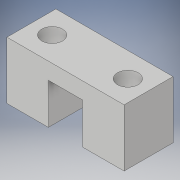
# Autodesk Inventor part: motor mount
Saved by Autodesk Inventor 2018 (Build 220112000, 112)
## iProperties
Created: 2019-04-09
Part Number: motor mount
Material: Generic
Document SubType Name: Modeling
Designer: Jayden
Density: 1 g/cm^3
Appearance: Default
Author: Jayden
Autodesk Inventor part; units mm, degrees
ref_plane "YZ Plane" through (0, 0, 0) normal (1, 0, 0) x (0, 1, 0)
ref_plane "XZ Plane" through (0, 0, 0) normal (0, 1, 0) x (-1, 0, 0)
ref_plane "XY Plane" through (0, 0, 0) normal (0, 0, 1) x (1, 0, 0)
sketch "Sketch1" plane through (0, 0, 0) normal (0, 0, 1) x (1, 0, 0)
  line L0 (-4.3614, 7.1036) -> (6.1386, 7.1036)
  line L1 (6.1386, 7.1036) -> (6.1386, -5.3964)
  line L2 (-4.3614, -5.3964) -> (-4.3614, 7.1036)
  line L3 (-4.3614, -5.3964) -> (-17.0614, -5.3964)
  line L4 (-4.3614, -5.3964) -> (8.3386, -5.3964) construction
  line L5 (-17.0614, -5.3964) -> (-17.0614, 12.1836)
  line L6 (-17.0614, 12.1836) -> (18.8386, 12.1836)
  line L7 (18.8386, 12.1836) -> (18.8386, -5.3964)
  line L8 (18.8386, -5.3964) -> (6.1386, -5.3964)
  point P0 (0, 0)
  dimension "d0" = 10.5
  dimension "d1" = 12.5
  dimension "d2" = 12.7
  dimension "d3" = 180
  dimension "d6" = 12.7
  dimension "d9" = 5.08
  constraints: 18 end point, 3 horizontal, 3 perpendicular, 2 parallel, 1 collinear, 1 point on line, 1 vertical
  measures "d0" distance of L1.end L2.start
  measures "d1" distance of L0.end L1.end
  measures "d2" distance of L2.start L3.end
  measures "d3" angle of L3 L4
  measures "d6" distance of L7.end L1.end
  measures "d9" distance between parallel lines of L6 L0
extrude "Extrusion1" add sketch "Sketch1" along normal blind 15
sketch "Sketch2" plane through (6.1386, -5.3964, 0) normal (0, -1, 0) x (1, 0, 0)
  circle A0 centre (6.35, 7.5) radius 3.175
  circle A1 centre (-16.85, 7.5) radius 3.175
  line L0 (0, 0) -> (12.7, 0) projected
  line L1 (-23.2, 0) -> (-23.2, 15) projected
  line L2 (-23.2, 15) -> (-10.5, 15) projected
  point P0 (-6.1386, 0)
  dimension "d12" = 6.35
  dimension "d13" = 6.35
  dimension "d14" = 7.5
  dimension "d15" = 6.35
  dimension "d16" = 6.35
  dimension "d17" = 7.5
  constraints: 2 centre point
  measures "d12" diameter of A0
  measures "d13" diameter of A1
  measures "d14" distance from line of L0 A0.centre
  measures "d15" horizontal distance of L0.start A0.centre
  measures "d16" distance from line of L1 A1.centre
  measures "d17" distance from line of L2 A1.centre
extrude "Extrusion2" cut sketch "Sketch2" against normal blind 21.5125
body "Solid1"
